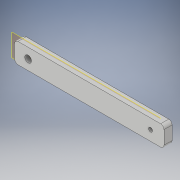
# Autodesk Inventor part: Fourbar-Rocker
Saved by Autodesk Inventor 2019 (Build 230136000, 136)
## iProperties
Created: 2021-06-06
Part Number: Fourbar-Rocker
Material: Generic
Document SubType Name: Modeling
Designer: micha
Density: 1 g/cm^3
Appearance: Default
Author: micha
Autodesk Inventor part; units mm, degrees
ref_plane "YZ Plane" through (0, 0, 0) normal (1, 0, 0) x (0, 1, 0)
ref_plane "XZ Plane" through (0, 0, 0) normal (0, 1, 0) x (-1, 0, 0)
ref_plane "XY Plane" through (0, 0, 0) normal (0, 0, 1) x (1, 0, 0)
sketch "Sketch1" plane through (0, 0, 0) normal (0, 0, 1) x (1, 0, 0)
  line L0 (0, 0) -> (221.6, 0)
  line L1 (221.6, 0) -> (221.6, 30)
  line L2 (221.6, 30) -> (0, 30)
  line L3 (0, 30) -> (0, 0)
  dimension "d0" = 221.6
  dimension "d1" = 30
  constraints: 8 end point, 2 parallel, 1 horizontal, 1 perpendicular
  measures "d0" distance of L2.end L1.end
  measures "d1" distance of L1.end L0.end
extrude "Extrusion1" add sketch "Sketch1" along normal blind 12
fillet "Fillet1" radius 5 4 edges at (0, 30, 6) (0, 0, 6) (221.6, 0, 6) (221.6, 30, 6)
sketch "Sketch2" plane through (0, 0, 12) normal (0, 0, 1) x (1, 0, 0)
  line L0 (0, 25) -> (0, 5) projected
  line L1 (0, 15) -> (20, 15)
  circle A0 centre (20, 15) radius 5
  line L2 (5, 0) -> (216.6, 0) projected
  line L3 (110.8, 0) -> (110.8, 30)
  line L4 (216.6, 30) -> (5, 30) projected
  line L5 (221.6, 5) -> (221.6, 25) projected
  line L6 (221.6, 15) -> (201.6, 15)
  circle A1 centre (201.6, 15) radius 3
  point P0 (0, 0)
  dimension "d5" = 20
  dimension "d6" = 10
  dimension "d9" = 20
  dimension "d10" = 6
  constraints: 6 end point, 4 midpoint, 2 centre point, 2 coincident, 2 horizontal
  measures "d5" distance of L1.start L1.end
  measures "d6" diameter of A0
  measures "d9" distance of L6.start L6.end
  measures "d10" diameter of A1
extrude "Extrusion2" cut sketch "Sketch2" against normal through all
ref_plane "Work Plane1" through (0, 0, 6) normal (0, 0, 1) x (1, 0, 0)
body "Solid1"
